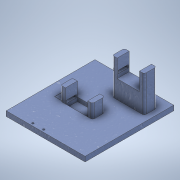
# Autodesk Inventor part: Base
Saved by Autodesk Inventor 2022 (Build 260153000, 153)
## iProperties
Created: 2021-11-09
Part Number: Base
Material: Generic
Document SubType Name: Modeling
Designer: Juan
Density: 1 g/cm^3
Appearance: Default
Author: Juan
Autodesk Inventor part; units mm, degrees
ref_plane "YZ Plane" through (0, 0, 0) normal (1, 0, 0) x (0, 1, 0)
ref_plane "XZ Plane" through (0, 0, 0) normal (0, 1, 0) x (-1, 0, 0)
ref_plane "XY Plane" through (0, 0, 0) normal (0, 0, 1) x (1, 0, 0)
sketch "Sketch1" plane through (0, 0, 0) normal (0, 1, 0) x (-1, 0, 0)
  line L0 (-30, -40) -> (-30, 40)
  line L1 (-30, 40) -> (30, 40)
  line L2 (30, 40) -> (30, -40)
  line L3 (30, -40) -> (-30, -40)
  line L4 (-30, -40) -> (30, 40) construction
  line L5 (-30, 40) -> (30, -40) construction
  point P0 (0, 0)
  dimension "d0" = 80
  dimension "d1" = 60
  constraints: 12 end point, 2 midpoint, 2 parallel, 1 perpendicular, 1 vertical
  measures "d0" distance of L0.start L0.end
  measures "d1" distance of L0.end L1.end
extrude "Extrusion1" add sketch "Sketch1" along normal blind 5
sketch "Sketch2" plane through (0, 5, 0) normal (0, 1, 0) x (1, 0, 0)
  circle A0 centre (-5.5, -37.5) radius 1
  circle A1 centre (5.5, -37.5) radius 1
  line L0 (-30, -40) -> (30, -40) projected
  line L1 (30, -40) -> (30, 40) projected
  point P0 (0, 0)
  dimension "d4" = 2
  dimension "d5" = 2
  dimension "d6" = 11
  dimension "d7" = 2.5
  dimension "d8" = 2.5
  dimension "d9" = 24.5
  constraints: 2 centre point
  measures "d4" diameter of A0
  measures "d5" diameter of A1
  measures "d6" distance of A1.centre A0.centre
  measures "d7" distance from line of L0 A0.centre
  measures "d8" distance from line of L0 A1.centre
  measures "d9" distance from line of L1 A1.centre
extrude "Extrusion2" cut sketch "Sketch2" against normal blind 4
sketch "Sketch3" plane through (0, 5, 0) normal (0, 1, 0) x (1, 0, 0)
  line L0 (30, -40) -> (30, 40) projected
  line L1 (30, -40) -> (0, -40)
  line L2 (-30, -40) -> (30, -40) projected
  line L3 (0, -40) -> (0, 2.107)
  line L4 (0, 2.107) -> (-6, 2.107)
  line L5 (-6, 2.107) -> (-6, 8.207)
  line L6 (-6, 8.207) -> (16.75, 8.207)
  line L7 (16.75, 8.207) -> (16.75, -3.993)
  line L8 (16.75, -3.993) -> (-6, -3.993)
  line L9 (-6, -3.993) -> (-6, 8.207)
  point P0 (0, 0)
  dimension "d12" = 42.107
  dimension "d13" = 6
  dimension "d14" = 6.1
  dimension "d15" = 22.75
  dimension "d16" = 12.2
  constraints: 16 end point, 3 perpendicular, 2 horizontal, 2 parallel, 1 midpoint
  measures "d12" distance of L1.end L3.end
  measures "d13" distance of L3.end L4.end
  measures "d14" distance of L4.end L5.end
  measures "d15" distance of L7.end L8.end
  measures "d16" distance of L6.end L7.end
extrude "Extrusion3" cut sketch "Sketch3" against normal blind 3.915
sketch "Sketch4" plane through (30, 0, 40) normal (1, 0, 0) x (0, 0, -1)
  line L0 (0, 0) -> (80, 0) projected
  line L1 (0, 5) -> (80, 5)
  line L2 (80, 5) -> (80, 0)
  line L3 (80, 0) -> (0, 0)
  line L4 (0, 0) -> (0, 5)
  point P0 (40, 0)
  constraints: 8 end point, 2 parallel, 1 horizontal, 1 perpendicular
extrude "Extrusion4" add sketch "Sketch4" along normal blind 20
sketch "Sketch5" plane through (-30, 0, -40) normal (0, 0, -1) x (-1, 0, 0)
  line L0 (0, 5) -> (-80, 5) projected
  line L1 (0, 0) -> (0, 5) projected
  line L2 (-80, 5) -> (0, 5)
  line L3 (0, 5) -> (0, 0)
  line L4 (0, 0) -> (-80, 0)
  line L5 (-80, 0) -> (-80, 5)
  point P0 (-30, 0)
  constraints: 8 end point, 2 parallel, 1 horizontal, 1 perpendicular
extrude "Extrusion5" add sketch "Sketch5" along normal blind 10
sketch "Sketch6" plane through (0, 5, 0) normal (0, 1, 0) x (1, 0, 0)
  line L0 (-30, -40) -> (-30, 50) projected
  line L1 (-30, -40) -> (0, -40)
  line L2 (-30, -40) -> (50, -40) projected
  line L3 (0, -40) -> (0, 32.107)
  line L4 (0, 32.107) -> (22.5, 32.107)
  line L5 (22.5, 32.107) -> (16.5, 32.107)
  line L6 (16.5, 32.107) -> (16.5, 38.207)
  line L7 (16.5, 38.207) -> (39.25, 38.207)
  line L8 (39.25, 38.207) -> (39.25, 26.007)
  line L9 (39.25, 26.007) -> (16.5, 26.007)
  line L10 (16.5, 26.007) -> (16.5, 38.207)
  point P0 (0, 0)
  dimension "d23" = 30
  dimension "d24" = 72.107
  dimension "d25" = 22.5
  dimension "d26" = 6
  dimension "d27" = 6.1
  dimension "d28" = 22.75
  dimension "d29" = 12.2
  constraints: 18 end point, 3 perpendicular, 2 horizontal, 2 parallel, 2 point on line
  measures "d23" distance of L0.start L1.end
  measures "d24" distance of L1.end L3.end
  measures "d25" distance of L3.end L4.end
  measures "d26" distance of L4.end L5.end
  measures "d27" distance of L5.end L6.end
  measures "d28" distance of L8.end L9.end
  measures "d29" distance of L7.end L8.end
extrude "Extrusion6" add sketch "Sketch6" along normal blind 18.52
sketch "Sketch7" plane through (0, 5, 0) normal (0, 1, 0) x (1, 0, 0)
  line L0 (16.75, 8.207) -> (16.75, -3.993) projected
  line L1 (16.75, -3.993) -> (21.625, -3.993)
  line L2 (21.625, -3.993) -> (21.625, 8.207)
  line L3 (21.625, 8.207) -> (16.75, 8.207)
  line L4 (16.75, 8.207) -> (16.75, -3.993)
  line L5 (-6, -3.993) -> (-6, 8.207) projected
  line L6 (-6, -3.993) -> (-10.875, -3.993)
  line L7 (-10.875, -3.993) -> (-10.875, 8.207)
  line L8 (-10.875, 8.207) -> (-6, 8.207)
  line L9 (-6, 8.207) -> (-6, -3.993)
  point P0 (0, 0)
  dimension "d32" = 4.875
  dimension "d33" = 4.875
  dimension "d34" = 12.2
  constraints: 16 end point, 4 parallel, 2 horizontal, 2 perpendicular
  measures "d32" distance of L3.end L2.end
  measures "d33" distance of L7.end L8.end
  measures "d34" distance of L6.end L7.end
extrude "Extrusion7" add sketch "Sketch7" along normal blind 14.135
sketch "Sketch8" plane through (-6, 1.085, 3.993) normal (1, 0, 0) x (0, 0, -1)
  line L0 (0, 0) -> (12.2, 0) projected
  line L1 (6.1, 0) -> (6.1, 3.8)
  line L2 (6.1, 3.8) -> (11.1, 3.8)
  line L3 (11.1, 3.8) -> (1.1, 3.8)
  line L4 (1.1, 3.8) -> (1.1, 6.8)
  line L5 (1.1, 6.8) -> (11.1, 6.8)
  line L6 (11.1, 6.8) -> (11.1, 3.8)
  point P0 (3.993, -1.085)
  dimension "d37" = 3.8
  dimension "d38" = 5
  dimension "d39" = 10
  dimension "d40" = 3
  constraints: 12 end point, 2 parallel, 2 perpendicular, 1 horizontal, 1 midpoint, 1 vertical
  measures "d37" distance of L1.start L1.end
  measures "d38" distance of L1.end L2.end
  measures "d39" distance of L4.end L5.end
  measures "d40" distance of L3.end L4.end
extrude "Extrusion8" cut sketch "Sketch8" against normal blind 12
sketch "Sketch9" plane through (0, 5, 0) normal (0, 1, 0) x (1, 0, 0)
  line L0 (16.5, 26.007) -> (16.5, 38.207) projected
  line L1 (16.5, 26.007) -> (11.625, 26.007)
  line L2 (11.625, 26.007) -> (11.625, 38.207)
  line L3 (11.625, 38.207) -> (16.5, 38.207)
  line L4 (16.5, 38.207) -> (16.5, 26.007)
  line L5 (39.25, 26.007) -> (16.5, 26.007) projected
  line L6 (39.25, 26.007) -> (44.125, 26.007)
  line L7 (44.125, 26.007) -> (44.125, 38.207)
  line L8 (44.125, 38.207) -> (39.25, 38.207)
  line L9 (39.25, 38.207) -> (39.25, 26.007)
  point P0 (0, 0)
  dimension "d43" = 4.875
  dimension "d44" = 12.2
  dimension "d45" = 4.875
  dimension "d46" = 12.2
  constraints: 16 end point, 4 parallel, 2 horizontal, 2 perpendicular
  measures "d43" distance of L2.end L3.end
  measures "d44" distance of L1.end L2.end
  measures "d45" distance of L8.end L7.end
  measures "d46" distance of L7.end L6.end
extrude "Extrusion9" add sketch "Sketch9" along normal blind 36.57
sketch "Sketch10" plane through (16.5, 23.52, -38.207) normal (1, 0, 0) x (0, 0, -1)
  line L0 (0, 0) -> (-12.2, 0) projected
  line L1 (-6.1, 0) -> (-6.1, 3.8)
  line L2 (-6.1, 3.8) -> (-1.1, 3.8)
  line L3 (-1.1, 3.8) -> (-11.1, 3.8)
  line L4 (-11.1, 3.8) -> (-11.1, 6.8)
  line L5 (-11.1, 6.8) -> (-1.1, 6.8)
  line L6 (-1.1, 6.8) -> (-1.1, 3.8)
  point P0 (-38.207, -23.52)
  point P1 (-6.1, 3.8)
  dimension "d49" = 3.8
  dimension "d50" = 5
  dimension "d51" = 10
  dimension "d52" = 3
  constraints: 12 end point, 2 parallel, 2 perpendicular, 1 horizontal, 1 midpoint, 1 vertical
  measures "d49" distance of L1.start L1.end
  measures "d50" distance of L1.end L2.end
  measures "d51" distance of L4.end L5.end
  measures "d52" distance of L3.end L4.end
extrude "Extrusion10" cut sketch "Sketch10" against normal up to surface (4.875 mm away)
fillet "Fillet1" radius 2 8 edges at (21.625, 12.0675, 3.993) (21.625, 12.0675, -8.207) (-10.875, 12.0675, 3.993) (-10.875, 12.0675, -8.207) (11.625, 23.285, -38.207) (11.625, 23.285, -26.007) (44.125, 23.285, -26.007) (44.125, 23.285, -38.207)
body "Solid1"
